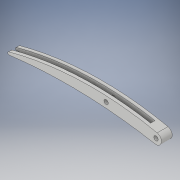
# Autodesk Inventor part: termite_beest_draft
Saved by Autodesk Inventor 2017 (Build 210142000, 142)
## iProperties
Created: 2016-08-26
Part Number: termite_beest_draft
Material: Generic
Document SubType Name: Modeling
Designer: Nic
Density: 1 g/cm^3
Appearance: Default
Author: Nic
Autodesk Inventor part; units mm, degrees
ref_plane "Work Plane1" through (0, 0, 0.75) normal (0, 0, 1) x (1, 0, 0)
ref_plane "YZ Plane" through (0, 0, 0) normal (1, 0, 0) x (0, 1, 0)
ref_plane "XZ Plane" through (0, 0, 0) normal (0, 1, 0) x (-1, 0, 0)
sketch "Sketch1" plane through (0, 0, 0) normal (0, 0, 1) x (1, 0, 0)
  circle A0 centre (68, 0) radius 1
  circle A1 centre (44.8999, 3) radius 1
  circle A2 centre (44.8999, 3) radius 2.5 construction
  arc A3 (-0.157, 0.5791) -> (0.0755, -0.5952) centre (0, 0) ccw
  arc A4 (68.5222, 2.4449) -> (-0.157, 0.5791) centre (38.035, -140.2958) ccw
  arc A5 (67.5488, -2.459) -> (0.0755, -0.5952) centre (27.8029, -219.0832) ccw
  arc A6 (67.5488, -2.459) -> (68.5222, 2.4449) centre (68, 0) ccw
  arc A7 (42.8188, 4.3853) -> (9.2918, 1.5821) centre (38.035, -140.2958) ccw
  arc A8 (42.6764, 1.8571) -> (9.2918, 1.5821) centre (27.8029, -219.0832) ccw
  arc A9 (42.8188, 4.3853) -> (42.6764, 1.8571) centre (44.8999, 3) ccw
  point P0 (44.8999, 6.5)
  dimension "d1" = 2
  dimension "d2" = 2
  dimension "d4" = 3
  dimension "d8" = 5
  dimension "d9" = 3.5
  dimension "d21" = 0.6
  dimension "d22" = 2.5
  dimension "d23" = 0
  dimension "d24" = 1.2
  dimension "d25" = 1.2
  dimension "d30" = 45
  dimension "d31" = 68
  constraints: 16 point on circle, 10 centre point, 6 tangent, 4 coincident, 2 concentric, 1 vertical alignment
  measures "d1" diameter of A0
  measures "d2" diameter of A1
  measures "d4" vertical distance of A0.centre A1.centre
  measures "d8" diameter of A2
  measures "d9" distance of A1.centre point (44.9, 6.5)
  measures "d21" radius of A3
  measures "d22" radius of A6
  measures "d23" vertical distance of point (0, 0) A0.centre
  measures "d24" radial gap between concentric circles of A5 A8
  measures "d25" radial gap between concentric circles of A4 A7
  measures "d30" distance of point (0, 0) A1.centre
  measures "d31" distance of A0.centre point (0, 0)
extrude "Extrusion1" add sketch "Sketch1" along normal blind 5 contours A4 A6 A5 A3 | A9 A8 A7
sketch "Sketch3" plane through (0, 0, 0) normal (0, 1, 0) x (-1, 0, 0)
  line L0 (4, 1.5) -> (-64, 1.5)
  line L1 (-64, 1.5) -> (-64, 3.5)
  line L2 (-64, 3.5) -> (4, 3.5)
  line L3 (4, 3.5) -> (4, 1.5)
  line L4 (-0.0755, 0) -> (-0.0755, 5) projected
  point P0 (0, 0)
  dimension "d34" = 1.5
  dimension "d35" = 4
  dimension "d36" = 2
  dimension "d37" = 68
  constraints: 8 end point, 2 parallel, 1 horizontal, 1 perpendicular
  measures "d34" distance from line of L0 point (0, 0)
  measures "d35" distance from line of L3 point (0, 0)
  measures "d36" distance between parallel lines of L2 L0
  measures "d37" distance from line of L2.end L1
extrude "Extrusion3" cut sketch "Sketch3" along normal through all both and the other way through all
body "Solid1"
